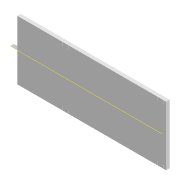
# Autodesk Inventor part: 00_Baseplate_Simmo_side3_v2
Saved by Autodesk Inventor 2022 (Build 260153000, 153)
## iProperties
Created: 2022-08-04
Part Number: 00_Baseplate_Simmo_side3_v2
Material: Generic
Document SubType Name: Modeling
Designer: wanghaoran
Density: 1 g/cm^3
Appearance: Default
Author: wanghaoran
Autodesk Inventor part; units mm, degrees
ref_plane "YZ Plane" through (0, 0, 0) normal (1, 0, 0) x (0, 1, 0)
ref_plane "XZ Plane" through (0, 0, 0) normal (0, 1, 0) x (-1, 0, 0)
ref_plane "XY Plane" through (0, 0, 0) normal (0, 0, 1) x (1, 0, 0)
sketch "Sketch3" plane through (0, 0, 0) normal (0, 0, 1) x (1, 0, 0)
  line L0 (0.8003, 0) -> (0.8003, 6) projected
  line L1 (0.8003, 0) -> (0.8003, -73) projected
  line L2 (-244.2385, 0) -> (-244.2385, 6) projected
  line L3 (0.8003, 6) -> (-250, 6)
  line L4 (-250, 6) -> (-250, -94)
  line L5 (-250, -94) -> (0.8003, -94)
  line L6 (0.8003, -94) -> (0.8003, 6)
  line L7 (-250, 0) -> (-250, 6) projected
  line L8 (8.2163, 0) -> (8.2163, -86) projected
  line L9 (8.2163, 0) -> (0.8003, 0)
  line L10 (0.8003, 0) -> (0.8003, -94)
  line L11 (0.8003, -94) -> (8.2163, -94)
  line L12 (8.2163, -94) -> (8.2163, 0)
  point P0 (0, 0)
  point P1 (-244.2385, 6)
  point P2 (-231.8779, 0)
  dimension "d10" = 100
  constraints: 16 end point, 4 parallel, 2 horizontal, 2 perpendicular
  measures "d10" distance of L3.end L4.end
extrude "Extrusion3" add sketch "Sketch3" along normal blind 6
sketch "Sketch4" plane through (0, 0, 6) normal (0, 0, 1) x (1, 0, 0)
  line L0 (0.8003, 6) -> (-250, 6) projected
  line L1 (-230, 0) -> (-230, 6) projected
  line L2 (-240, 6) -> (-230, 6) projected
  line L3 (-240, 6) -> (-240, 0) projected
  line L4 (-240, 0) -> (-230, 0) projected
  line L5 (-230, 0) -> (-229.9, 0)
  line L6 (-229.9, 0) -> (-229.9, 6)
  line L7 (-229.9, 6) -> (-230, 6)
  line L8 (-230, 6) -> (-230, 0)
  line L9 (-240, 0) -> (-240.1, 0)
  line L10 (-240.1, 0) -> (-240.1, 6)
  line L11 (-240.1, 6) -> (-240, 6)
  line L12 (-240, 6) -> (-240, 0)
  point P0 (0, 0)
  dimension "d20" = 0.1
  dimension "d21" = 6
  dimension "d22" = 0.1
  dimension "d23" = 6
  constraints: 16 end point, 4 parallel, 2 horizontal, 2 perpendicular
  measures "d20" distance of L7.end L6.end
  measures "d21" distance of L6.end L5.end
  measures "d22" distance of L10.end L11.end
  measures "d23" distance of L9.end L10.end
extrude "Extrusion4" cut sketch "Sketch4" against normal blind 6
pattern_linear "Rectangular Pattern2" count 12 spacing 20 along (1, 0, 0) of "Extrusion4"
ref_plane "Work Plane2" through (-250, -44, 0) normal (0, -1, 0) x (1, 0, 0)
mirror "Mirror2" about plane through (-250, -44, 0) normal (0, -1, 0) of "Extrusion4", "Rectangular Pattern2"
sketch "Sketch5" plane through (0, 0, 6) normal (0, 0, 1) x (1, 0, 0)
  line L0 (-212.25, -5.4) -> (-217.75, -5.4)
  line L1 (-217.75, -5.4) -> (-217.75, -3)
  line L2 (-217.75, -3) -> (-212.25, -3)
  line L3 (-212.25, -3) -> (-212.25, -5.4)
  line L4 (-209.9, 6) -> (-209.9, 0) projected
  line L5 (-209.9, 0) -> (-220.1, 0) projected
  point P0 (0, 0)
  dimension "d26" = 5.5
  dimension "d27" = 2.4
  dimension "d28" = 2.35
  dimension "d29" = 3
  constraints: 8 end point, 2 parallel, 1 horizontal, 1 perpendicular
  measures "d26" distance of L1.end L2.end
  measures "d27" distance of L0.end L1.end
  measures "d28" distance between parallel lines of L4 L3
  measures "d29" distance between parallel lines of L5 L2
extrude "Extrusion5" cut sketch "Sketch5" against normal blind 6
pattern_linear "Rectangular Pattern3" count 3 spacing 100 along (1, 0, 0) count 2 spacing 79.6 along (0, -1, 0) of "Extrusion5"
body "Solid2"
